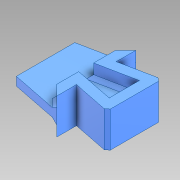
# Autodesk Inventor part: StraightRais-215
Saved by Autodesk Inventor 2021 (Build 250183000, 183)
## iProperties
Created: 2021-02-11
Part Number: StraightRais-215
Material: ABS プラスチック
Document SubType Name: Modeling
Designer: kumagai
Density: 1.06 g/cm^3
Appearance: 滑らか - 青
cp: 0.000 mm
ConnectorLength: 15.000 mm
RailWidth: 38.000 mm
JointFH: 9.500 mm
PrinterOffset: 0.000 mm
StraightLength: 215.000 mm
OuterWall: 2.000 mm
InnerWall: 2.400 mm
InsideWidth: 18.600 mm
RailHeight: 8.400 mm
RailDepth: 3.200 mm
JointMW1: 13.000 mm
JointMW2: 9.400 mm
JointMH: 9.000 mm
JointFW1: 13.300 mm
JointFW2: 9.600 mm
SupportGap: 0.200 mm
SupportRib: 0.500 mm
Author: kumagai
Autodesk Inventor part; units mm, degrees
ref_plane "YZ Plane" through (0, 0, 0) normal (1, 0, 0) x (0, 1, 0)
ref_plane "XZ Plane" through (0, 0, 0) normal (0, 1, 0) x (-1, 0, 0)
ref_plane "XY Plane" through (0, 0, 0) normal (0, 0, 1) x (1, 0, 0)
sketch "スケッチ1" plane through (0, 0, 0) normal (0, 1, 0) x (-1, 0, 0)
  line L0 (0, -13.02) -> (0, 13.02) projected
  line L1 (-13.2, 0) -> (16.2, 0) projected
  line L2 (0, -4.7) -> (-9, -6.5)
  line L3 (-9, -6.5) -> (-9, 6.5)
  line L4 (-9, 6.5) -> (0, 4.7)
  line L5 (0, -9.3) -> (0, -4.7)
  line L6 (0, 4.7) -> (0, 9.3)
  line L7 (2.4, -1.7725) -> (-6.6, -3.5725)
  line L8 (-6.6, -3.5725) -> (-6.6, 3.5725)
  line L9 (-6.6, 3.5725) -> (2.4, 1.7725)
  line L10 (2.4, -6.9) -> (2.4, -1.7725)
  line L11 (2.4, 1.7725) -> (2.4, 6.9)
  line L12 (2.4, -6.9) -> (0, -9.3)
  line L13 (2.4, 6.9) -> (0, 9.3)
  line L14 (12, -6.9) -> (12, 6.9)
  line L15 (12, 6.9) -> (0, 9.3)
  line L16 (12, -6.9) -> (0, -9.3)
  point P0 (0, 0)
  point P1 (0, 9.3)
  point P2 (0, -9.3)
  dimension "d2" = 9
  dimension "d3" = 13
  dimension "d5" = 9.4
  dimension "d13" = 2.4
  dimension "d14" = 2.4
  dimension "d15" = 2.4
  dimension "d24" = 2.4
  dimension "d63" = 2.4
  dimension "d64" = 18.6
  dimension "d65" = 12
  dimension "d74" = 18.6
  dimension "d75" = 2.4
  constraints: 30 end point, 3 collinear, 3 parallel, 2 point on line, 2 vertical, 3 other
  measures "d2" distance between parallel lines of L3 L5
  measures "d3" distance of L3.end L2.end
  measures "d5" distance of L4.end L2.start
  measures "d13" distance between parallel lines of L5 L10
  measures "d14" distance between parallel lines of L3 L8
  measures "d15" distance between parallel lines of L4 L9
  measures "d24" distance between parallel lines of L7 L2
  measures "d63" horizontal distance of L12.end L10.start
  measures "d64" distance of L13.end L12.end
  measures "d65" distance between parallel lines of L14 L0
  measures "d74" distance of L5.start L6.end
  measures "d75" vertical distance of L14.end L6.end
extrude "押し出し2" add sketch "スケッチ1" along normal blind 3.2 and the other way blind 5.2 contours L0 L7 L10 L12 | L2 L3 L1 L8 L7 L0 | L3 L4 L0 L9 L8 L1 | L0 L13 L11 L9
extrude "押し出し1" add sketch "スケッチ1" against normal blind 2
chamfer "面取り4" distance 0.8 angle 45 2 edges at (9, -1, 6.5) (9, -1, -6.5)
chamfer "面取り5" distance 0.8 angle 45 14 edges at (2.1, 0, -2.6725) (6.6, 0, 0) (-2.4, 0, -4.3362) (2.1, 0, 2.6725) (-2.4, 0, 4.3362) (-1.2, 0, 8.1) (-1.2, 0, -8.1) (-1.2, -2, 8.1) (-2.4, -2, 4.3362) (2.1, -2, 2.6725) (6.6, -2, 0) (2.1, -2, -2.6725) (-2.4, -2, -4.3362) (-1.2, -2, -8.1)
equation "\"d2\" = JointMH"
equation "\"d3\" = JointMW1 - 2 * cp"
equation "\"d5\" = JointMW2 - 2 * cp"
equation "\"d13\" = InnerWall"
equation "\"d14\" = InnerWall"
equation "\"d15\" = InnerWall"
equation "\"d24\" = InnerWall"
equation "\"rib\" = 0.5"
equation "\"gap\" = 0.2"
equation "\"JointMH\" = 9"
equation "\"JointMW1\" = 13"
equation "\"cp\" = 0"
equation "\"JointMW2\" = 9.4"
equation "\"InnerWall\" = 2.4"
